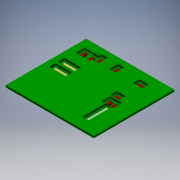
# Autodesk Inventor part: gora
Saved by Autodesk Inventor 2016 SP1 (Build 200210100, 210)
## iProperties
Created: 2019-02-13
Part Number: gora
Material: Ogólny
Document SubType Name: Modeling
Designer: Maciek
Density: 1 g/cm^3
Appearance: Zarys tablicy
Author: Maciek
Autodesk Inventor part; units mm, degrees
ref_plane "YZ Plane" through (0, 0, 0) normal (1, 0, 0) x (0, 1, 0)
ref_plane "XZ Plane" through (0, 0, 0) normal (0, 1, 0) x (-1, 0, 0)
ref_plane "XY Plane" through (0, 0, 0) normal (0, 0, 1) x (1, 0, 0)
sketch "Szkic1" plane through (0, 0, 0) normal (0, 0, 1) x (1, 0, 0)
  line L0 (30, 28) -> (93, 28)
  line L1 (93, 28) -> (93, 85)
  line L2 (93, 85) -> (30, 85)
  line L3 (30, 85) -> (30, 28)
  circle A0 centre (34, 64) radius 0.5
  circle A1 centre (37, 64) radius 0.5
  circle A2 centre (39, 64) radius 0.5
  circle A3 centre (42, 64) radius 0.5
  circle A4 centre (34, 57) radius 0.5
  circle A5 centre (37, 57) radius 0.5
  circle A6 centre (39, 57) radius 0.5
  circle A7 centre (42, 57) radius 0.5
  circle A8 centre (66, 35) radius 0.5
  circle A9 centre (66, 38) radius 0.5
  circle A10 centre (66, 40) radius 0.5
  circle A11 centre (66, 43) radius 0.5
  circle A12 centre (66, 45) radius 0.5
  circle A13 centre (66, 48) radius 0.5
  circle A14 centre (41, 76) radius 0.5
  circle A15 centre (41, 79) radius 0.5
  circle A16 centre (35, 76) radius 0.5
  circle A17 centre (35, 79) radius 0.5
  circle A18 centre (59, 79) radius 0.5
  circle A19 centre (59, 81) radius 0.5
  circle A20 centre (76, 35) radius 0.5
  circle A21 centre (76, 38) radius 0.5
  circle A22 centre (76, 40) radius 0.5
  circle A23 centre (76, 43) radius 0.5
  circle A24 centre (76, 45) radius 0.5
  circle A25 centre (76, 48) radius 0.5
  circle A26 centre (53, 79) radius 0.5
  circle A27 centre (53, 81) radius 0.5
  circle A28 centre (78, 57) radius 0.5
  circle A29 centre (78, 54) radius 0.5
  circle A30 centre (46, 79) radius 0.5
  circle A31 centre (46, 81) radius 0.5
  circle A32 centre (39, 36) radius 0.5
  circle A33 centre (37, 36) radius 0.5
  circle A34 centre (82, 57) radius 0.5
  circle A35 centre (82, 54) radius 0.5
  circle A36 centre (42, 52) radius 0.5
  circle A37 centre (39, 52) radius 0.5
  circle A38 centre (37, 52) radius 0.5
  circle A39 centre (42, 47) radius 0.5
  circle A40 centre (39, 47) radius 0.5
  circle A41 centre (37, 47) radius 0.5
  circle A42 centre (42, 41) radius 0.5
  circle A43 centre (39, 41) radius 0.5
  circle A44 centre (37, 41) radius 0.5
  circle A45 centre (80, 79) radius 0.5
  circle A46 centre (77, 79) radius 0.5
  circle A47 centre (79, 62) radius 0.5
  circle A48 centre (76, 62) radius 0.5
  circle A49 centre (81, 35) radius 0.5
  circle A50 centre (81, 38) radius 0.5
  circle A51 centre (81, 40) radius 0.5
  circle A52 centre (81, 43) radius 0.5
  circle A53 centre (81, 45) radius 0.5
  circle A54 centre (81, 48) radius 0.5
  circle A55 centre (81, 50) radius 0.5
  constraints: 56 centre point, 8 end point
extrude "schemat.brd_Kontur" add sketch "Szkic1" along normal blind 1
sketch "C050-030X075, C050-030X075_1" plane through (0, 0, 1) normal (0, 0, 1) x (1, 0, 0)
  line L0 (62, 52) -> (62, 58)
  line L1 (62, 58) -> (64, 58)
  line L2 (64, 58) -> (64, 52)
  line L3 (64, 52) -> (62, 52)
  constraints: 8 end point
extrude "C1_2" add sketch "C050-030X075, C050-030X075_1" along normal blind 1
sketch "C025-030X050, C025-030X050_3" plane through (0, 0, 1) normal (0, 0, 1) x (1, 0, 0)
  line L0 (66, 55) -> (66, 59)
  line L1 (66, 59) -> (68, 59)
  line L2 (68, 59) -> (68, 55)
  line L3 (68, 55) -> (66, 55)
  constraints: 8 end point
extrude "C2_4" add sketch "C025-030X050, C025-030X050_3" along normal blind 1
sketch "C025-030X050, C025-030X050_5" plane through (0, 0, 1) normal (0, 0, 1) x (1, 0, 0)
  line L0 (49, 59) -> (49, 55)
  line L1 (49, 55) -> (47, 55)
  line L2 (47, 55) -> (47, 59)
  line L3 (47, 59) -> (49, 59)
  constraints: 8 end point
extrude "C3_6" add sketch "C025-030X050, C025-030X050_5" along normal blind 1
sketch "C025-030X050, C025-030X050_7" plane through (0, 0, 1) normal (0, 0, 1) x (1, 0, 0)
  line L0 (68, 77) -> (68, 81)
  line L1 (68, 81) -> (70, 81)
  line L2 (70, 81) -> (70, 77)
  line L3 (70, 77) -> (68, 77)
  constraints: 8 end point
extrude "C4_8" add sketch "C025-030X050, C025-030X050_7" along normal blind 1
sketch "C025-030X050, C025-030X050_9" plane through (0, 0, 1) normal (0, 0, 1) x (1, 0, 0)
  line L0 (88, 57) -> (88, 53)
  line L1 (88, 53) -> (86, 53)
  line L2 (86, 53) -> (86, 57)
  line L3 (86, 57) -> (88, 57)
  constraints: 8 end point
extrude "C5_10" add sketch "C025-030X050, C025-030X050_9" along normal blind 1
sketch "E2_5-5, E2_5-5_11" plane through (0, 0, 1) normal (0, 0, 1) x (1, 0, 0)
  line L0 (71, 77) -> (71, 81)
  line L1 (71, 81) -> (75, 81)
  line L2 (75, 81) -> (75, 77)
  line L3 (75, 77) -> (71, 77)
  constraints: 8 end point
extrude "C6_12" add sketch "E2_5-5, E2_5-5_11" along normal blind 1
sketch "E2_5-5, E2_5-5_13" plane through (0, 0, 1) normal (0, 0, 1) x (1, 0, 0)
  line L0 (85, 63) -> (89, 63)
  line L1 (89, 63) -> (89, 59)
  line L2 (89, 59) -> (85, 59)
  line L3 (85, 59) -> (85, 63)
  constraints: 8 end point
extrude "C7_14" add sketch "E2_5-5, E2_5-5_13" along normal blind 1
sketch "1X04, 1X04_15" plane through (0, 0, 1) normal (0, 0, 1) x (1, 0, 0)
  line L0 (33, 65) -> (43, 65)
  line L1 (43, 65) -> (43, 63)
  line L2 (43, 63) -> (33, 63)
  line L3 (33, 63) -> (33, 65)
  constraints: 8 end point
extrude "ENKODER1_16" add sketch "1X04, 1X04_15" along normal blind 1
sketch "1X04, 1X04_17" plane through (0, 0, 1) normal (0, 0, 1) x (1, 0, 0)
  line L0 (33, 58) -> (43, 58)
  line L1 (43, 58) -> (43, 56)
  line L2 (43, 56) -> (33, 56)
  line L3 (33, 56) -> (33, 58)
  constraints: 8 end point
extrude "ENKODER2_18" add sketch "1X04, 1X04_17" along normal blind 1
sketch "1X06, 1X06_19" plane through (0, 0, 1) normal (0, 0, 1) x (1, 0, 0)
  line L0 (65, 34) -> (65, 48)
  line L1 (65, 48) -> (67, 48)
  line L2 (67, 48) -> (67, 34)
  line L3 (67, 34) -> (65, 34)
  constraints: 8 end point
extrude "HV_20" add sketch "1X06, 1X06_19" along normal blind 1
sketch "DIL28-3, MEGA8-P_21" plane through (0, 0, 1) normal (0, 0, 1) x (1, 0, 0)
  line L0 (57, 75) -> (57, 39)
  line L1 (57, 39) -> (53, 39)
  line L2 (53, 39) -> (53, 75)
  line L3 (53, 75) -> (57, 75)
  constraints: 8 end point
extrude "IC1_22" add sketch "DIL28-3, MEGA8-P_21" along normal blind 1
sketch "DIL16, L293D_23" plane through (0, 0, 1) normal (0, 0, 1) x (1, 0, 0)
  line L0 (88, 68) -> (68, 68)
  line L1 (68, 68) -> (68, 72)
  line L2 (68, 72) -> (88, 72)
  line L3 (88, 72) -> (88, 68)
  constraints: 8 end point
extrude "IC2_24" add sketch "DIL16, L293D_23" along normal blind 1
sketch "0204_7, 0204_7_25" plane through (0, 0, 1) normal (0, 0, 1) x (1, 0, 0)
  line L0 (73, 52) -> (66, 52)
  line L1 (66, 52) -> (66, 54)
  line L2 (66, 54) -> (73, 54)
  line L3 (73, 54) -> (73, 52)
  constraints: 8 end point
extrude "L1_26" add sketch "0204_7, 0204_7_25" along normal blind 1
sketch "1X02, 1X02_27" plane through (0, 0, 1) normal (0, 0, 1) x (1, 0, 0)
  line L0 (40, 76) -> (40, 80)
  line L1 (40, 80) -> (42, 80)
  line L2 (42, 80) -> (42, 76)
  line L3 (42, 76) -> (40, 76)
  constraints: 8 end point
extrude "LED1_28" add sketch "1X02, 1X02_27" along normal blind 1
sketch "1X02, 1X02_29" plane through (0, 0, 1) normal (0, 0, 1) x (1, 0, 0)
  line L0 (34, 76) -> (34, 80)
  line L1 (34, 80) -> (36, 80)
  line L2 (36, 80) -> (36, 76)
  line L3 (36, 76) -> (34, 76)
  constraints: 8 end point
extrude "LED2_30" add sketch "1X02, 1X02_29" along normal blind 1
sketch "1X02, 1X02_31" plane through (0, 0, 1) normal (0, 0, 1) x (1, 0, 0)
  line L0 (58, 78) -> (58, 82)
  line L1 (58, 82) -> (60, 82)
  line L2 (60, 82) -> (60, 78)
  line L3 (60, 78) -> (58, 78)
  constraints: 8 end point
extrude "LIPOL_32" add sketch "1X02, 1X02_31" along normal blind 1
sketch "1X06, 1X06_33" plane through (0, 0, 1) normal (0, 0, 1) x (1, 0, 0)
  line L0 (75, 34) -> (75, 48)
  line L1 (75, 48) -> (77, 48)
  line L2 (77, 48) -> (77, 34)
  line L3 (77, 34) -> (75, 34)
  constraints: 8 end point
extrude "LV_34" add sketch "1X06, 1X06_33" along normal blind 1
sketch "1X02, 1X02_35" plane through (0, 0, 1) normal (0, 0, 1) x (1, 0, 0)
  line L0 (52, 78) -> (52, 82)
  line L1 (52, 82) -> (54, 82)
  line L2 (54, 82) -> (54, 78)
  line L3 (54, 78) -> (52, 78)
  constraints: 8 end point
extrude "P-EL-IN_36" add sketch "1X02, 1X02_35" along normal blind 1
sketch "1X02, 1X02_37" plane through (0, 0, 1) normal (0, 0, 1) x (1, 0, 0)
  line L0 (79, 57) -> (79, 53)
  line L1 (79, 53) -> (77, 53)
  line L2 (77, 53) -> (77, 57)
  line L3 (77, 57) -> (79, 57)
  constraints: 8 end point
extrude "P-EL-OUT_38" add sketch "1X02, 1X02_37" along normal blind 1
sketch "1X02, 1X02_39" plane through (0, 0, 1) normal (0, 0, 1) x (1, 0, 0)
  line L0 (45, 78) -> (45, 82)
  line L1 (45, 82) -> (47, 82)
  line L2 (47, 82) -> (47, 78)
  line L3 (47, 78) -> (45, 78)
  constraints: 8 end point
extrude "P-S-IN_40" add sketch "1X02, 1X02_39" along normal blind 1
sketch "1X02, 1X02_41" plane through (0, 0, 1) normal (0, 0, 1) x (1, 0, 0)
  line L0 (40, 35) -> (36, 35)
  line L1 (36, 35) -> (36, 37)
  line L2 (36, 37) -> (40, 37)
  line L3 (40, 37) -> (40, 35)
  constraints: 8 end point
extrude "P-S-OUT_42" add sketch "1X02, 1X02_41" along normal blind 1
sketch "0204_7, 0204_7_43" plane through (0, 0, 1) normal (0, 0, 1) x (1, 0, 0)
  line L0 (47, 68) -> (47, 75)
  line L1 (47, 75) -> (49, 75)
  line L2 (49, 75) -> (49, 68)
  line L3 (49, 68) -> (47, 68)
  constraints: 8 end point
extrude "R1_44" add sketch "0204_7, 0204_7_43" along normal blind 1
sketch "0204_7, 0204_7_45" plane through (0, 0, 1) normal (0, 0, 1) x (1, 0, 0)
  line L0 (64, 81) -> (64, 74)
  line L1 (64, 74) -> (62, 74)
  line L2 (62, 74) -> (62, 81)
  line L3 (62, 81) -> (64, 81)
  constraints: 8 end point
extrude "R3_46" add sketch "0204_7, 0204_7_45" along normal blind 1
sketch "0204_7, 0204_7_47" plane through (0, 0, 1) normal (0, 0, 1) x (1, 0, 0)
  line L0 (64, 71) -> (64, 78)
  line L1 (64, 78) -> (66, 78)
  line L2 (66, 78) -> (66, 71)
  line L3 (66, 71) -> (64, 71)
  constraints: 8 end point
extrude "R4_48" add sketch "0204_7, 0204_7_47" along normal blind 1
sketch "0204_7, 0204_7_49" plane through (0, 0, 1) normal (0, 0, 1) x (1, 0, 0)
  line L0 (45, 72) -> (38, 72)
  line L1 (38, 72) -> (38, 74)
  line L2 (38, 74) -> (45, 74)
  line L3 (45, 74) -> (45, 72)
  constraints: 8 end point
extrude "R5_50" add sketch "0204_7, 0204_7_49" along normal blind 1
sketch "0204_7, 0204_7_51" plane through (0, 0, 1) normal (0, 0, 1) x (1, 0, 0)
  line L0 (45, 69) -> (38, 69)
  line L1 (38, 69) -> (38, 71)
  line L2 (38, 71) -> (45, 71)
  line L3 (45, 71) -> (45, 69)
  constraints: 8 end point
extrude "R6_52" add sketch "0204_7, 0204_7_51" along normal blind 1
sketch "1X02, 1X02_53" plane through (0, 0, 1) normal (0, 0, 1) x (1, 0, 0)
  line L0 (83, 57) -> (83, 53)
  line L1 (83, 53) -> (81, 53)
  line L2 (81, 53) -> (81, 57)
  line L3 (81, 57) -> (83, 57)
  constraints: 8 end point
extrude "RASPBERRY_54" add sketch "1X02, 1X02_53" along normal blind 1
sketch "1X03, 1X03_55" plane through (0, 0, 1) normal (0, 0, 1) x (1, 0, 0)
  line L0 (42, 51) -> (36, 51)
  line L1 (36, 51) -> (36, 53)
  line L2 (36, 53) -> (42, 53)
  line L3 (42, 53) -> (42, 51)
  constraints: 8 end point
extrude "SERWO1_56" add sketch "1X03, 1X03_55" along normal blind 1
sketch "1X03, 1X03_57" plane through (0, 0, 1) normal (0, 0, 1) x (1, 0, 0)
  line L0 (42, 46) -> (36, 46)
  line L1 (36, 46) -> (36, 48)
  line L2 (36, 48) -> (42, 48)
  line L3 (42, 48) -> (42, 46)
  constraints: 8 end point
extrude "SERWO2_58" add sketch "1X03, 1X03_57" along normal blind 1
sketch "1X03, 1X03_59" plane through (0, 0, 1) normal (0, 0, 1) x (1, 0, 0)
  line L0 (42, 40) -> (36, 40)
  line L1 (36, 40) -> (36, 42)
  line L2 (36, 42) -> (42, 42)
  line L3 (42, 42) -> (42, 40)
  constraints: 8 end point
extrude "SERWO3_60" add sketch "1X03, 1X03_59" along normal blind 1
sketch "1X02, 1X02_61" plane through (0, 0, 1) normal (0, 0, 1) x (1, 0, 0)
  line L0 (81, 78) -> (77, 78)
  line L1 (77, 78) -> (77, 80)
  line L2 (77, 80) -> (81, 80)
  line L3 (81, 80) -> (81, 78)
  constraints: 8 end point
extrude "SILNIK1_62" add sketch "1X02, 1X02_61" along normal blind 1
sketch "1X02, 1X02_63" plane through (0, 0, 1) normal (0, 0, 1) x (1, 0, 0)
  line L0 (80, 61) -> (76, 61)
  line L1 (76, 61) -> (76, 63)
  line L2 (76, 63) -> (80, 63)
  line L3 (80, 63) -> (80, 61)
  constraints: 8 end point
extrude "SILNIK2_64" add sketch "1X02, 1X02_63" along normal blind 1
sketch "1X07, 1X07_65" plane through (0, 0, 1) normal (0, 0, 1) x (1, 0, 0)
  line L0 (80, 35) -> (80, 51)
  line L1 (80, 51) -> (82, 51)
  line L2 (82, 51) -> (82, 35)
  line L3 (82, 35) -> (80, 35)
  constraints: 8 end point
extrude "SPI_66" add sketch "1X07, 1X07_65" along normal blind 1
sketch "Szkic35" plane through (0, 0, 2) normal (0, 0, 1) x (1, 0, 0)
  line L0 (93, 28) -> (93, 85) construction
  line L1 (93, 85) -> (96, 85) construction
  line L2 (96, 85) -> (96, 88) construction
  line L3 (30, 28) -> (30, 25) construction
  line L4 (30, 25) -> (27, 25) construction
  line L5 (96, 88) -> (27, 88)
  line L6 (27, 88) -> (27, 25)
  line L7 (27, 25) -> (96, 25)
  line L8 (96, 25) -> (96, 88)
  line L9 (43, 58) -> (33, 58) construction
  line L10 (33, 58) -> (31.5, 58) construction
  line L11 (30, 85) -> (30, 28) construction
  line L12 (31.5, 58) -> (31.5, 59.5) construction
  line L13 (33, 56) -> (43, 56) construction
  line L14 (43, 56) -> (43, 54.5) construction
  line L15 (43, 54.5) -> (44.5, 54.5) construction
  line L16 (31.5, 59.5) -> (44.5, 59.5)
  line L17 (44.5, 59.5) -> (44.5, 54.5)
  line L18 (44.5, 54.5) -> (31.5, 54.5)
  line L19 (31.5, 54.5) -> (31.5, 59.5)
  line L20 (33, 65) -> (31.5, 65) construction
  line L21 (31.5, 65) -> (31.5, 66.5) construction
  line L22 (43, 63) -> (33, 63) construction
  line L23 (43, 63) -> (43, 61.5) construction
  line L24 (43, 61.5) -> (44.5, 61.5) construction
  line L25 (31.5, 66.5) -> (44.5, 66.5)
  line L26 (44.5, 66.5) -> (44.5, 61.5)
  line L27 (44.5, 61.5) -> (31.5, 61.5)
  line L28 (31.5, 61.5) -> (31.5, 66.5)
  line L29 (45, 78) -> (45, 82) construction
  line L30 (45, 82) -> (45, 83.5) construction
  line L31 (45, 83.5) -> (43.5, 83.5) construction
  line L32 (42, 80) -> (42, 76) construction
  line L33 (42, 80) -> (42, 81.5) construction
  line L34 (42, 81.5) -> (36.1129, 81.5) construction
  line L35 (34, 80) -> (36, 80) construction
  line L36 (34, 80) -> (32.5, 80) construction
  line L37 (32.5, 80) -> (32.5, 81.5) construction
  line L38 (34, 76) -> (34, 80) construction
  line L39 (34, 76) -> (34, 74.5) construction
  line L40 (34, 74.5) -> (32.5, 74.5) construction
  line L41 (47, 82) -> (47, 78) construction
  line L42 (47, 82) -> (48.5, 82) construction
  line L43 (48.5, 82) -> (48.5, 83.5) construction
  line L44 (42, 76) -> (43.5, 76) construction
  line L45 (43.5, 76) -> (43.5, 74.5) construction
  line L46 (47, 78) -> (48.5, 78) construction
  line L47 (48.5, 78) -> (48.5, 76.5) construction
  line L48 (36.1129, 81.5) -> (32.5, 81.5)
  line L49 (32.5, 81.5) -> (32.5, 74.5)
  line L50 (32.5, 74.5) -> (43.5, 74.5)
  line L51 (48.5, 76.5) -> (43.5, 76.5)
  line L52 (43.5, 76.5) -> (43.5, 74.5)
  line L53 (48.5, 76.5) -> (48.5, 83.5)
  line L54 (48.5, 83.5) -> (43.5, 83.5)
  line L55 (36, 81.5) -> (42, 81.5)
  line L56 (42, 81.5) -> (36.1129, 81.5)
  line L57 (42, 81.5) -> (43.5, 81.5)
  line L58 (43.5, 81.5) -> (43.5, 83.5)
  line L59 (52, 82) -> (54, 82) construction
  line L60 (52, 82) -> (52, 83.5) construction
  line L61 (52, 83.5) -> (50.5, 83.5) construction
  line L62 (60, 82) -> (60, 78) construction
  line L63 (60, 78) -> (61.5, 78) construction
  line L64 (61.5, 78) -> (61.5, 76.5) construction
  line L65 (58, 78) -> (58, 82) construction
  line L66 (58, 82) -> (56.5, 82) construction
  line L67 (56.5, 82) -> (56.5, 83.5) construction
  line L68 (56.5, 83.5) -> (61.5, 83.5)
  line L69 (61.5, 83.5) -> (61.5, 76.5)
  line L70 (61.5, 76.5) -> (56.5, 76.5)
  line L71 (56.5, 76.5) -> (56.5, 83.5)
  line L72 (77, 80) -> (81, 80) construction
  line L73 (77, 80) -> (77, 81.5) construction
  line L74 (77, 81.5) -> (75.5, 81.5) construction
  line L75 (81, 78) -> (77, 78) construction
  line L76 (81, 78) -> (82.5, 78) construction
  line L77 (82.5, 78) -> (82.5, 76.5) construction
  line L78 (80, 63) -> (76, 63) construction
  line L79 (76, 63) -> (76, 64.5) construction
  line L80 (76, 64.5) -> (74.5, 64.5) construction
  line L81 (76, 61) -> (80, 61) construction
  line L82 (80, 61) -> (80, 59.5) construction
  line L83 (80, 59.5) -> (81.5, 59.5) construction
  line L84 (77, 57) -> (77.5, 57) construction
  line L85 (77, 57) -> (75.5, 57) construction
  line L86 (75.5, 57) -> (75.5, 58.5) construction
  line L87 (77, 53) -> (77, 57) construction
  line L88 (77, 53) -> (75.5, 53) construction
  line L89 (75.5, 53) -> (75.5, 51.5) construction
  line L90 (82, 51) -> (80, 51) construction
  line L91 (80, 51) -> (78.5, 51) construction
  line L92 (80, 51) -> (80, 35) construction
  line L93 (80, 35) -> (78.5, 35) construction
  line L94 (78.5, 35) -> (78.5, 33.5) construction
  line L95 (82, 35) -> (81.5, 35) construction
  line L96 (82, 35) -> (83.5, 35) construction
  line L97 (83.5, 35) -> (83.5, 33.5) construction
  line L98 (83, 53) -> (81, 53) construction
  line L99 (83, 53) -> (84.5, 53) construction
  line L100 (84.5, 53) -> (84.5, 51.5) construction
  line L101 (83, 57) -> (83, 53) construction
  line L102 (83, 57) -> (84.5, 57) construction
  line L103 (84.5, 57) -> (84.5, 58.5) construction
  line L104 (75.5, 58.5) -> (75.5, 51.5)
  line L105 (75.5, 51.5) -> (78.5, 51.5)
  line L106 (78.5, 51.5) -> (78.5, 33.5)
  line L107 (78.5, 33.5) -> (83.5, 33.5)
  line L108 (83.5, 33.5) -> (83.5, 51.5)
  line L109 (83.5, 51.5) -> (84.5, 51.5)
  line L110 (85, 59) -> (85, 63) projected
  line L111 (84.5, 51.5) -> (84.5, 58.5)
  line L112 (84.5, 58.5) -> (75.5, 58.5)
  line L113 (74.5, 64.5) -> (81.5, 64.5)
  line L114 (81.5, 64.5) -> (81.5, 59.5)
  line L115 (81.5, 59.5) -> (74.5, 59.5)
  line L116 (74.5, 59.5) -> (74.5, 64.5)
  line L117 (75.5, 81.5) -> (82.5, 81.5)
  line L118 (82.5, 81.5) -> (82.5, 76.5)
  line L119 (82.5, 76.5) -> (75.5, 76.5)
  line L120 (75.5, 76.5) -> (75.5, 81.5)
  point P0 (0, 0)
  dimension "d69" = 3
  dimension "d70" = 3
  dimension "d71" = 3
  dimension "d72" = 3
  dimension "d73" = 1.5
  dimension "d74" = 1.5
  dimension "d75" = 1.5
  dimension "d76" = 1.5
  dimension "d77" = 1.5
  dimension "d78" = 1.5
  dimension "d79" = 1.5
  dimension "d80" = 1.5
  dimension "d81" = 1.5
  dimension "d82" = 1.5
  dimension "d83" = 1.5
  dimension "d84" = 1.5
  dimension "d85" = 1.5
  dimension "d86" = 1.5
  dimension "d87" = 1.5
  dimension "d88" = 1.5
  dimension "d89" = 1.5
  dimension "d90" = 1.5
  dimension "d91" = 1.5
  dimension "d92" = 1.5
  dimension "d93" = 1.5
  dimension "d94" = 1.5
  dimension "d95" = 1.5
  dimension "d96" = 1.5
  dimension "d97" = 1.5
  dimension "d98" = 1.5
  dimension "d99" = 1.5
  dimension "d100" = 1.5
  dimension "d101" = 1.5
  dimension "d102" = 1.5
  dimension "d103" = 1.5
  dimension "d104" = 1.5
  dimension "d105" = 1.5
  dimension "d106" = 1.5
  dimension "d107" = 1.5
  dimension "d108" = 1.5
  dimension "d109" = 1.5
  dimension "d110" = 1.5
  dimension "d111" = 1.5
  dimension "d112" = 1.5
  dimension "d113" = 1.5
  dimension "d114" = 1.5
  dimension "d115" = 1.5
  dimension "d116" = 1.5
  dimension "d117" = 1.5
  dimension "d118" = 1.5
  dimension "d119" = 1.5
  dimension "d120" = 1.5
  constraints: 192 end point, 38 perpendicular, 25 horizontal, 12 parallel, 10 vertical, 2 point on line
  measures "d69" distance of L0.end L1.end
  measures "d70" distance of L1.end L2.end
  measures "d71" distance of L3.start L3.end
  measures "d72" distance of L3.end L4.end
  measures "d73" distance of L9.end L10.end
  measures "d74" distance of L10.end L12.end
  measures "d75" distance of L13.end L14.end
  measures "d76" distance of L14.end L15.end
  measures "d77" distance of L20.start L20.end
  measures "d78" distance of L20.end L21.end
  measures "d79" distance of L22.start L23.end
  measures "d80" distance of L23.end L24.end
  measures "d81" distance of L29.end L30.end
  measures "d82" distance of L30.end L31.end
  measures "d83" distance of L32.start L33.end
  measures "d84" distance of L35.start L36.end
  measures "d85" distance of L36.end L37.end
  measures "d86" distance of L38.start L39.end
  measures "d87" distance of L39.end L40.end
  measures "d88" distance of L41.start L42.end
  measures "d89" distance of L42.end L43.end
  measures "d90" distance of L32.end L44.end
  measures "d91" distance of L44.end L45.end
  measures "d92" distance of L41.end L46.end
  measures "d93" distance of L46.end L47.end
  measures "d94" distance of L59.start L60.end
  measures "d95" distance of L60.end L61.end
  measures "d96" distance of L62.end L63.end
  measures "d97" distance of L63.end L64.end
  measures "d98" distance of L65.end L66.end
  measures "d99" distance of L66.end L67.end
  measures "d100" distance of L72.start L73.end
  measures "d101" distance of L73.end L74.end
  measures "d102" distance of L75.start L76.end
  measures "d103" distance of L76.end L77.end
  measures "d104" distance of L78.end L79.end
  measures "d105" distance of L79.end L80.end
  measures "d106" distance of L81.end L82.end
  measures "d107" distance of L82.end L83.end
  measures "d108" distance of L84.start L85.end
  measures "d109" distance of L85.end L86.end
  measures "d110" distance of L87.start L88.end
  measures "d111" distance of L88.end L89.end
  measures "d112" distance of L90.end L91.end
  measures "d113" distance of L92.end L93.end
  measures "d114" distance of L93.end L94.end
  measures "d115" distance of L95.start L96.end
  measures "d116" distance of L96.end L97.end
  measures "d117" distance of L98.start L99.end
  measures "d118" distance of L99.end L100.end
  measures "d119" distance of L101.start L102.end
  measures "d120" distance of L102.end L103.end
extrude "Wyciągnięcie proste35" add sketch "Szkic35" along normal blind 1.5
